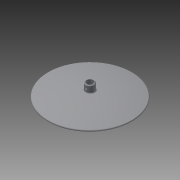
# Autodesk Inventor part: Launcher
Saved by Autodesk Inventor 2014 (Build 180170000, 170)
## iProperties
Created: 2014-01-06
Part Number: Launcher
Material: Generic
Document SubType Name: Modeling
Designer: Andrew Toennies
Density: 1 g/cm^3
Appearance: Default
Author: Andrew Toennies
Autodesk Inventor part; units mm, degrees
ref_plane "YZ Plane" through (0, 0, 0) normal (1, 0, 0) x (0, 1, 0)
sketch "Sketch1" plane through (0, 0, 0) normal (0, 0, 1) x (1, 0, 0)
  arc A0 (61.8921, 298.45) -> (-61.8921, 298.45) centre (0, 0) ccw
  line L0 (-61.8921, 298.45) -> (61.8921, 298.45)
  arc A1 (87.9882, 298.45) -> (-87.9882, 298.45) centre (0, 0) ccw
  line L1 (-61.8921, 298.45) -> (-87.9882, 298.45)
  line L2 (61.8921, 298.45) -> (87.9882, 298.45)
  line L3 (0, 311.15) -> (0, 304.8)
  dimension "d0" = 609.6
  dimension "d1" = 298.45
  dimension "d2" = 6.35
  constraints: 8 end point, 6 point on circle, 2 centre point, 2 horizontal, 1 coincident, 1 collinear
  measures "d0" diameter of A0
  measures "d1" distance from line of A0.centre L0
  measures "d2" radial gap between concentric circles of A0 A1
revolve "Revolution1" add sketch "Sketch1" angle 360 about axis through (0, 311.15, 0) along (0, -1, 0) contours A0 L3 A1 L2
fillet "Fillet1" radius 127 1 edges at (-61.8921, 298.45, 0)
fillet "Fillet2" radius 1.5875 1 edges at (-87.9882, 298.45, 0)
ref_plane "Work Plane1" through (0, 311.15, 0) normal (0, 1, 0) x (-1, 0, 0)
sketch "Sketch2" plane through (0, 311.15, 0) normal (0, 1, 0) x (-1, 0, 0)
  circle A0 centre (0, 0) radius 6.35
  circle A1 centre (0, 0) radius 7.9375
  dimension "d6" = 12.7
  dimension "d7" = 15.875
  constraints: 2 centre point, 2 coincident
  measures "d6" diameter of A0
  measures "d7" diameter of A1
extrude "Extrusion1" add sketch "Sketch2" along normal blind 12.7 and the other way blind 2.54
ref_plane "Work Plane2" through (0, 311.15, 7.9375) normal (0, 0, 1) x (1, 0, 0)
fillet "Fillet3" radius 1.5875 3 edges at (7.9375, 323.85, 0) (0.0002, 311.0487, 7.9375) (0, 311.0487, -7.9375)
sketch "Sketch3" plane through (0, 311.15, 7.9375) normal (0, 0, 1) x (1, 0, 0)
  circle A0 centre (0, 6.35) radius 1.5875
  line L0 (0, 6.35) -> (0, -311.15) construction
  dimension "d12" = 3.175
  dimension "d13" = 317.5
  constraints: 2 end point, 1 centre point, 1 vertical
  measures "d12" diameter of A0
  measures "d13" distance of L0.end L0.start
extrude "Extrusion2" cut sketch "Sketch3" against normal blind 25.4
body "Solid1"
